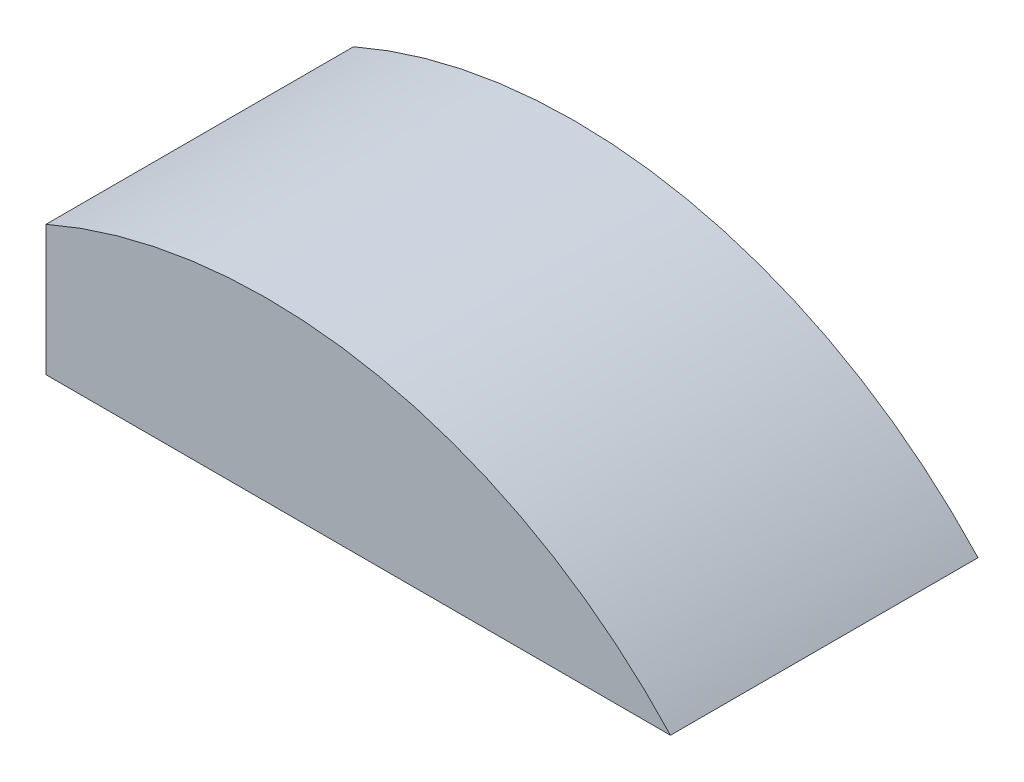
# Autodesk Inventor part: KB33-046-002-006 - Заглушка
Saved by Autodesk Inventor 2020 (Build 240168000, 168)
## iProperties
Created: 2021-07-29
Part Number: KB33-046-002-006 - Заглушка
Material: Типовые
Document SubType Name: Modeling
Designer: Петров Иван
Mass: 2.46616 g
Surface Area: 12.6721 cm^2
Volume: 2.46616 cm^3
Density: 1 g/cm^3
Appearance: По умолчанию
Author: Петров Иван
Autodesk Inventor part; units mm, degrees
ref_plane "YZ Plane" through (0, 0, 0) normal (1, 0, 0) x (0, 1, 0)
ref_plane "XZ Plane" through (0, 0, 0) normal (0, 1, 0) x (-1, 0, 0)
ref_plane "XY Plane" through (0, 0, 0) normal (0, 0, 1) x (1, 0, 0)
sketch "Эскиз1" plane through (0, 0, 0) normal (0, 0, 1) x (1, 0, 0)
  arc A0 (28.4298, -5.9319) -> (0, 0) centre (10.0583, -22.8873) ccw
  line L0 (0, -5.9315) -> (0, 0)
  line L1 (23.9975, -5.9315) -> (0, -5.9315)
  line L2 (23.9975, -5.9315) -> (23.998, -5.9315)
  line L3 (23.998, -5.9319) -> (23.998, -5.9315)
  line L4 (23.998, -5.9319) -> (28.4298, -5.9319)
  point P0 (0, 0)
  point P1 (-10.0583, 22.8873)
  constraints: 10 end point, 2 point on circle, 1 centre point, 1 horizontal
extrude "Выдавливание1" add sketch "Эскиз1" along normal blind 14
